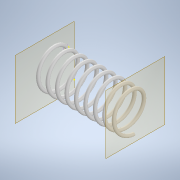
# Autodesk Inventor part: Coil
Saved by Autodesk Inventor 2022 (Build 260153000, 153)
## iProperties
Created: 2022-08-26
Part Number: Coil
Material: Generic
Document SubType Name: Modeling
Designer: David
Density: 1 g/cm^3
Appearance: Default
Author: David
Autodesk Inventor part; units mm, degrees
ref_plane "XZ Plane" through (0, 0, 0) normal (0, 1, 0) x (-1, 0, 0)
ref_plane "XY Plane" through (0, 0, 0) normal (0, 0, 1) x (1, 0, 0)
sketch "Sketch2" plane through (0, 0, 0) normal (0, 0, 1) x (1, 0, 0)
  line L0 (0, 0) -> (18.8807, 0)
  line L1 (18.8807, -5.5) -> (18.8807, 0)
  circle A0 centre (18.8807, -5.5) radius 0.5
  dimension "d11" = 18.8807
  dimension "d12" = 1
  dimension "d21" = 5.5
  constraints: 4 end point, 1 centre point, 1 coincident, 1 horizontal, 1 vertical
  measures "d11" distance of L0.start L0.end
  measures "d12" diameter of A0
  measures "d21" distance of L1.start L0.end
coil "Coil2" sketch "Sketch2" operation add axis through (0, 0, 0) along (-1, 0, 0) pitch 3 turns 8.666667 hand right
ref_plane "Work Plane1" through (19.3807, -5.5, 0) normal (1, 0, 0) x (0, 1, 0)
sketch "Sketch3" plane through (-7.1193, 2.75, -4.7631) normal (0, -0.866, -0.5) x (1, 0, 0)
  circle A0 centre (0, 0) radius 0.5 projected
  point P0 (7.1193, 5.5)
  point P1 (-0.5, 0)
  point P2 (0.5, 0)
  constraints: 1 point on circle
ref_plane "Work Plane2" through (-7.6193, 2.75, -4.7631) normal (1, 0, 0) x (0, 1, 0)
body "Solid2"
